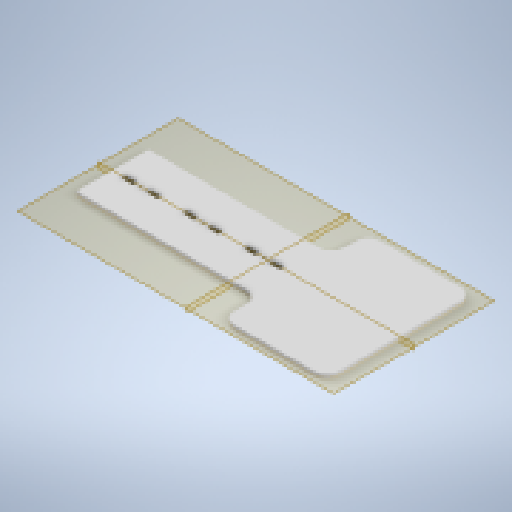
# Autodesk Inventor part: Крепление хвоста
Saved by Autodesk Inventor 2023.2 (Build 272271030, 271C)
## iProperties
Created: 2024-03-15
Part Number: Крепление хвоста
Material: Типовые
Document SubType Name: Modeling
Designer: I9232
Density: 1 g/cm^3
Appearance: По умолчанию
Author: I9232
Autodesk Inventor part; units mm, degrees
sketch "Эскиз1" plane through (0, 0, 0) normal (0, 1, 0) x (-1, 0, 0)
  line L0 (126.566, 29.5) -> (-22.5, 29.5)
  line L1 (-107.5, 29.5) -> (-107.5, -29.5)
  line L2 (-22.5, -29.5) -> (126.566, -29.5)
  line L3 (126.566, -29.5) -> (126.566, 29.5)
  line L4 (-22.5, 29.5) -> (-22.4506, 59.5)
  line L5 (-22.4506, 59.5) -> (-107.4506, 59.5)
  line L6 (-107.4506, 59.5) -> (-107.5, 29.5)
  line L7 (-22.5, -29.5) -> (-22.4506, -59.5)
  line L8 (-22.4506, -59.5) -> (-107.4506, -59.5)
  line L9 (-107.4506, -59.5) -> (-107.5, -29.5)
  point P0 (0, 0)
  dimension "d6" = 59
  dimension "d7" = 119
  dimension "d8" = 149.066
  dimension "d9" = 85
  dimension "d10" = 30
  constraints: 20 end point, 4 parallel, 3 equal length, 1 horizontal, 1 perpendicular, 1 vertical, 2 other
  measures "d6" distance of L2.end L0.start
  measures "d7" distance of L8.end L5.end
  measures "d8" distance of L0.start L0.end
  measures "d9" distance of L4.end L5.end
  measures "d10" distance of L0.end L4.end
extrude "Выдавливание1" add sketch "Эскиз1" along normal mid plane 4
fillet "Сопряжение1" radius 10 6 edges at (22.5, 0, -29.5) (22.4506, 0, -59.5) (22.4506, 0, 59.5) (107.4506, 0, -59.5) (107.4506, 0, 59.5) (22.5, 0, 29.5)
sketch "Эскиз2" plane through (0, -2, 0) normal (0, -1, 0) x (1, 0, 0)
  line L0 (-118.066, -2) -> (-108.066, -2) projected
  line L1 (-108.066, -2) -> (-108.066, 2) projected
  line L2 (-108.066, 2) -> (-118.066, 2) projected
  line L3 (-118.066, 2) -> (-118.066, -2) projected
  line L4 (-98.066, -2) -> (-88.066, -2) projected
  line L5 (-88.066, -2) -> (-88.066, 2) projected
  line L6 (-88.066, 2) -> (-98.066, 2) projected
  line L7 (-98.066, 2) -> (-98.066, -2) projected
  line L8 (-68.066, -2) -> (-58.066, -2) projected
  line L9 (-58.066, -2) -> (-58.066, 2) projected
  line L10 (-58.066, 2) -> (-68.066, 2) projected
  line L11 (-68.066, 2) -> (-68.066, -2) projected
  line L12 (-48.066, -2) -> (-38.066, -2) projected
  line L13 (-38.066, -2) -> (-38.066, 2) projected
  line L14 (-38.066, 2) -> (-48.066, 2) projected
  line L15 (-48.066, 2) -> (-48.066, -2) projected
  line L16 (-18.066, -2) -> (-8.066, -2) projected
  line L17 (-8.066, -2) -> (-8.066, 2) projected
  line L18 (-8.066, 2) -> (-18.066, 2) projected
  line L19 (-18.066, 2) -> (-18.066, -2) projected
  line L20 (1.934, -2) -> (11.934, -2) projected
  line L21 (11.934, -2) -> (11.934, 2) projected
  line L22 (11.934, 2) -> (1.934, 2) projected
  line L23 (1.934, 2) -> (1.934, -2) projected
  point P0 (0, 0)
extrude "Выдавливание2" cut sketch "Эскиз2" against normal up to surface (4 mm away)
sketch "Эскиз3" plane through (0, -2, 0) normal (0, -1, 0) x (1, 0, 0)
  line L0 (1.934, 2) -> (1.934, -2) projected
  line L1 (-8.066, -2) -> (-8.066, 2) projected
  line L2 (-48.066, 2) -> (-48.066, -2) projected
  line L3 (-58.066, -2) -> (-58.066, 2) projected
  line L4 (-98.066, 2) -> (-98.066, -2) projected
  line L5 (-108.066, -2) -> (-108.066, 2) projected
  circle A0 centre (-3.066, 0) radius 1.5
  circle A1 centre (-53.066, 0) radius 1.5
  circle A2 centre (-103.066, 0) radius 1.5
  line L6 (1.934, 2) -> (1.934, -2) projected
  line L7 (1.934, 0) -> (-8.066, 0) construction
  line L8 (-8.066, 2) -> (-8.066, -2) projected
  line L9 (-48.066, -2) -> (-48.066, 2) projected
  line L10 (-48.066, 0) -> (-58.066, 0) construction
  line L11 (-58.066, 2) -> (-58.066, -2) projected
  line L12 (-98.066, -2) -> (-98.066, 2) projected
  line L13 (-98.066, 0) -> (-108.066, 0) construction
  line L14 (-108.066, 2) -> (-108.066, -2) projected
  point P0 (0, 0)
  point P1 (-3.066, 0)
  point P2 (-53.066, 0)
  point P3 (-103.066, 0)
  dimension "d14" = 3
  constraints: 9 midpoint, 6 end point, 3 centre point, 3 coincident, 2 equal radius
  measures "d14" diameter of A0
extrude "Выдавливание3" cut sketch "Эскиз3" against normal up to surface (4 mm away)
sketch "Эскиз4" plane through (-126.566, -2, 29.5) normal (-1, 0, 0) x (0, 0, 1)
  line L0 (0, 4) -> (-59, 4) projected
  line L1 (-59, 0) -> (0, 0) projected
  line L2 (-54.5, 4) -> (-49.5, 4)
  line L3 (-49.5, 4) -> (-49.5, 0)
  line L4 (-49.5, 0) -> (-54.5, 0)
  line L5 (-54.5, 0) -> (-54.5, 4)
  line L6 (-59, 4) -> (-59, 0) projected
  line L7 (-39.5, 4) -> (-34.5, 4)
  line L8 (-34.5, 4) -> (-34.5, 0)
  line L9 (-34.5, 0) -> (-39.5, 0)
  line L10 (-39.5, 0) -> (-39.5, 4)
  line L11 (-24.5, 4) -> (-19.5, 4)
  line L12 (-19.5, 4) -> (-19.5, 0)
  line L13 (-19.5, 0) -> (-24.5, 0)
  line L14 (-24.5, 0) -> (-24.5, 4)
  line L15 (-9.5, 4) -> (-4.5, 4)
  line L16 (-4.5, 4) -> (-4.5, 0)
  line L17 (-4.5, 0) -> (-9.5, 0)
  line L18 (-9.5, 0) -> (-9.5, 4)
  point P0 (-29.5, 2)
  point P1 (-9.5, 0)
  point P2 (-24.5, 0)
  point P3 (-39.5, 0)
  point P4 (-54.5, 0)
  dimension "d17" = 5
  dimension "d18" = 4.5
  dimension "d19" = 10
  dimension "d20" = 5
  dimension "d23" = 30
  constraints: 32 end point, 4 parallel, 4 point on line, 3 horizontal, 2 perpendicular, 16 other
  measures "d17" distance of L2.end L2.start
  measures "d18" distance between parallel lines of L5 L6
  measures "d19" distance between parallel lines of L10 L3
  measures "d20" distance of L8.end L9.end
  measures "d23" distance of L2.start L11.start
extrude "Выдавливание4" add sketch "Эскиз4" along normal blind 3 contours L16 L1 L18 L0 | L12 L1 L14 L0 | L8 L1 L10 L0 | L3 L1 L5 L0
sketch "Эскиз5" plane through (-126.566, -2, -29.5) normal (0, 0, -1) x (-1, 0, 0)
  line L0 (0, 4) -> (-139.0495, 4) projected
  line L1 (-18.5, 0) -> (-8.5, 0) projected
  line L2 (-15, 4) -> (-5, 4)
  line L3 (-5, 4) -> (-5, 0)
  line L4 (-5, 0) -> (-15, 0)
  line L5 (-15, 0) -> (-15, 4)
  line L6 (0, 0) -> (-139.0495, 0) projected
  line L7 (-35, 4) -> (-25, 4)
  line L8 (-25, 4) -> (-25, 0)
  line L9 (-25, 0) -> (-35, 0)
  line L10 (-35, 0) -> (-35, 4)
  line L11 (0, 4) -> (0, 0) projected
  line L12 (-55, 4) -> (-45, 4)
  line L13 (-45, 4) -> (-45, 0)
  line L14 (-45, 0) -> (-55, 0)
  line L15 (-55, 0) -> (-55, 4)
  line L16 (-75, 4) -> (-65, 4)
  line L17 (-65, 4) -> (-65, 0)
  line L18 (-65, 0) -> (-75, 0)
  line L19 (-75, 0) -> (-75, 4)
  point P0 (-126.566, 2)
  point P1 (-15, 0)
  point P2 (-35, 0)
  point P3 (-55, 0)
  point P4 (-75, 0)
  dimension "d30" = 10
  dimension "d31" = 10
  dimension "d32" = 5
  dimension "d33" = 10
  dimension "d36" = 40
  constraints: 32 end point, 5 point on line, 4 parallel, 3 horizontal, 2 perpendicular, 16 other
  measures "d30" distance of L7.end L7.start
  measures "d31" distance of L2.end L2.start
  measures "d32" distance between parallel lines of L11 L3
  measures "d33" distance between parallel lines of L5 L8
  measures "d36" distance of L2.start L12.start
extrude "Выдавливание5" add sketch "Эскиз5" along normal blind 3 contours L3 L4 L1 L5 L0 | L8 L6 L10 L0 | L13 L6 L15 L0 | L17 L6 L19 L0
mirror "Зеркальное отражение1" about plane through (0, 0, 0) normal (0, 0, 1) of "Выдавливание5"
sketch "Эскиз6" plane through (0, -2, 0) normal (0, -1, 0) x (1, 0, 0)
  line L0 (93.0791, -30.9) -> (93.0791, -26.9) projected
  line L1 (93.0791, -26.9) -> (87.0791, -26.9) projected
  line L2 (87.0791, -26.9) -> (87.0791, -30.9) projected
  line L3 (87.0791, -30.9) -> (93.0791, -30.9) projected
  line L4 (93.0791, 30.9) -> (93.0791, 26.9) projected
  line L5 (87.0791, 30.9) -> (93.0791, 30.9) projected
  line L6 (87.0791, 26.9) -> (87.0791, 30.9) projected
  line L7 (93.0791, 26.9) -> (87.0791, 26.9) projected
  line L8 (71.0791, 30.9) -> (77.0791, 30.9) projected
  line L9 (77.0791, 30.9) -> (77.0791, 26.9) projected
  line L10 (77.0791, 26.9) -> (71.0791, 26.9) projected
  line L11 (71.0791, 26.9) -> (71.0791, 30.9) projected
  line L12 (58.5057, 30.9) -> (58.5057, 26.9) projected
  line L13 (58.5057, 26.9) -> (52.5057, 26.9) projected
  line L14 (52.5057, 30.9) -> (58.5057, 30.9) projected
  line L15 (52.5057, 26.9) -> (52.5057, 30.9) projected
  line L16 (42.5057, 30.9) -> (42.5057, 26.9) projected
  line L17 (42.5057, 26.9) -> (36.5057, 26.9) projected
  line L18 (36.5057, 26.9) -> (36.5057, 30.9) projected
  line L19 (36.5057, 30.9) -> (42.5057, 30.9) projected
  line L20 (77.0791, -26.9) -> (71.0791, -26.9) projected
  line L21 (71.0791, -30.9) -> (77.0791, -30.9) projected
  line L22 (77.0791, -30.9) -> (77.0791, -26.9) projected
  line L23 (71.0791, -26.9) -> (71.0791, -30.9) projected
  line L24 (58.5057, -30.9) -> (58.5057, -26.9) projected
  line L25 (52.5057, -30.9) -> (58.5057, -30.9) projected
  line L26 (58.5057, -26.9) -> (52.5057, -26.9) projected
  line L27 (52.5057, -26.9) -> (52.5057, -30.9) projected
  line L28 (42.5057, -30.9) -> (42.5057, -26.9) projected
  line L29 (36.5057, -30.9) -> (42.5057, -30.9) projected
  line L30 (42.5057, -26.9) -> (36.5057, -26.9) projected
  line L31 (36.5057, -26.9) -> (36.5057, -30.9) projected
  point P0 (0, 0)
extrude "Выдавливание6" cut sketch "Эскиз6" against normal up to surface (4 mm away)
sketch "Эскиз7" plane through (0, -2, 0) normal (0, -1, 0) x (1, 0, 0)
  point P0 (0, 0)
sketch "Эскиз8" plane through (0, -2, 0) normal (0, -1, 0) x (1, 0, 0)
  circle A0 centre (82.0791, -28.9) radius 1.5
  circle A1 centre (82.0791, 28.9) radius 1.5
  circle A2 centre (47.5057, 28.9) radius 1.5
  circle A3 centre (47.5057, -28.9) radius 1.5
  line L0 (52.5057, -30.9) -> (52.5057, -26.9) projected
  line L1 (42.5057, -26.9) -> (42.5057, -30.9) projected
  line L2 (77.0791, -26.9) -> (77.0791, -30.9) projected
  line L3 (87.0791, -26.9) -> (87.0791, -30.9) projected
  line L4 (87.0791, 26.9) -> (87.0791, 30.9) projected
  line L5 (77.0791, 30.9) -> (77.0791, 26.9) projected
  line L6 (52.5057, 26.9) -> (52.5057, 30.9) projected
  line L7 (42.5057, 30.9) -> (42.5057, 26.9) projected
  line L8 (87.0791, -26.9) -> (87.0791, -30.9) projected
  line L9 (87.0791, -28.9) -> (77.0791, -28.9) construction
  line L10 (77.0791, -30.9) -> (77.0791, -26.9) projected
  line L11 (52.5057, -28.9) -> (42.5057, -28.9) construction
  line L12 (87.0791, 26.9) -> (87.0791, 30.9) projected
  line L13 (87.0791, 28.9) -> (77.0791, 28.9) construction
  line L14 (52.5057, 28.9) -> (42.5057, 28.9) construction
  point P0 (0, 0)
  point P1 (82.0791, -28.9)
  point P2 (47.5057, 28.9)
  point P3 (82.0791, 28.9)
  dimension "d45" = 3
  constraints: 12 midpoint, 8 end point, 4 centre point, 4 coincident, 3 equal radius
  measures "d45" diameter of A0
extrude "Выдавливание7" cut sketch "Эскиз8" against normal up to surface (4 mm away)
sketch "Эскиз9" plane through (0, 2, 0) normal (0, 1, 0) x (1, 0, 0)
  line L0 (-108.016, -29.5) -> (-105.116, -29.5)
  line L1 (-105.116, -14.6) -> (-108.016, -14.6)
  line L2 (-111.566, -29.5) -> (-101.566, -29.5) projected
  line L3 (-103.766, -21.4) -> (-103.766, -19.6)
  line L4 (-109.366, -19.6) -> (-109.366, -21.4)
  line L5 (-106.566, -14.6) -> (-106.566, -29.5) construction
  line L6 (-108.016, -14.6) -> (-108.016, -19.6)
  line L7 (-108.016, -21.4) -> (-108.016, -29.5)
  line L8 (-109.366, -21.4) -> (-108.016, -21.4)
  line L9 (-105.116, -21.4) -> (-103.766, -21.4)
  line L10 (-103.766, -19.6) -> (-105.116, -19.6)
  line L11 (-108.016, -19.6) -> (-109.366, -19.6)
  line L12 (-105.116, -29.5) -> (-105.116, -21.4)
  line L13 (-105.116, -19.6) -> (-105.116, -14.6)
  line L14 (-68.016, -19.6) -> (-69.366, -19.6)
  line L15 (-68.016, -14.6) -> (-68.016, -19.6)
  line L16 (-65.116, -19.6) -> (-65.116, -14.6)
  line L17 (-65.116, -14.6) -> (-68.016, -14.6)
  line L18 (-69.366, -21.4) -> (-68.016, -21.4)
  line L19 (-69.366, -19.6) -> (-69.366, -21.4)
  line L20 (-63.766, -21.4) -> (-63.766, -19.6)
  line L21 (-65.116, -21.4) -> (-63.766, -21.4)
  line L22 (-66.566, -14.6) -> (-66.566, -29.5) construction
  line L23 (-68.016, -21.4) -> (-68.016, -29.5)
  line L24 (-65.116, -29.5) -> (-65.116, -21.4)
  line L25 (-68.016, -29.5) -> (-65.116, -29.5)
  line L26 (-63.766, -19.6) -> (-65.116, -19.6)
  line L27 (-94.5323, 0) -> (-86.001, 0) construction
  line L28 (-108.016, 29.5) -> (-105.116, 29.5)
  line L29 (-105.116, 14.6) -> (-108.016, 14.6)
  line L30 (-111.566, 29.5) -> (-101.566, 29.5)
  line L31 (-103.766, 21.4) -> (-103.766, 19.6)
  line L32 (-109.366, 19.6) -> (-109.366, 21.4)
  line L33 (-106.566, 14.6) -> (-106.566, 29.5) construction
  line L34 (-108.016, 14.6) -> (-108.016, 19.6)
  line L35 (-108.016, 21.4) -> (-108.016, 29.5)
  line L36 (-109.366, 21.4) -> (-108.016, 21.4)
  line L37 (-105.116, 21.4) -> (-103.766, 21.4)
  line L38 (-103.766, 19.6) -> (-105.116, 19.6)
  line L39 (-108.016, 19.6) -> (-109.366, 19.6)
  line L40 (-105.116, 29.5) -> (-105.116, 21.4)
  line L41 (-105.116, 19.6) -> (-105.116, 14.6)
  line L42 (-68.016, 19.6) -> (-69.366, 19.6)
  line L43 (-68.016, 14.6) -> (-68.016, 19.6)
  line L44 (-65.116, 19.6) -> (-65.116, 14.6)
  line L45 (-65.116, 14.6) -> (-68.016, 14.6)
  line L46 (-69.366, 21.4) -> (-68.016, 21.4)
  line L47 (-69.366, 19.6) -> (-69.366, 21.4)
  line L48 (-63.766, 21.4) -> (-63.766, 19.6)
  line L49 (-65.116, 21.4) -> (-63.766, 21.4)
  line L50 (-66.566, 14.6) -> (-66.566, 29.5) construction
  line L51 (-68.016, 21.4) -> (-68.016, 29.5)
  line L52 (-65.116, 29.5) -> (-65.116, 21.4)
  line L53 (-68.016, 29.5) -> (-65.116, 29.5)
  line L54 (-63.766, 19.6) -> (-65.116, 19.6)
  line L55 (-126.566, -10) -> (-126.566, -20) projected
  line L56 (-116.566, -16.45) -> (-116.566, -13.55)
  line L57 (-126.566, -13.55) -> (-126.566, -16.45)
  line L58 (-121.566, -17.8) -> (-119.766, -17.8)
  line L59 (-119.766, -12.2) -> (-121.566, -12.2)
  line L60 (-116.566, -15) -> (-126.566, -15) construction
  line L61 (-126.566, 10) -> (-126.566, 20)
  line L62 (-116.566, 16.45) -> (-116.566, 13.55)
  line L63 (-126.566, 13.55) -> (-126.566, 16.45)
  line L64 (-121.566, 17.8) -> (-119.766, 17.8)
  line L65 (-119.766, 12.2) -> (-121.566, 12.2)
  line L66 (-116.566, 15) -> (-126.566, 15) construction
  line L67 (-121.566, -12.2) -> (-121.566, -13.55)
  line L68 (-121.566, -16.45) -> (-121.566, -17.8)
  line L69 (-119.766, -17.8) -> (-119.766, -16.45)
  line L70 (-119.766, -13.55) -> (-119.766, -12.2)
  line L71 (-126.566, -16.45) -> (-121.566, -16.45)
  line L72 (-119.766, -16.45) -> (-116.566, -16.45)
  line L73 (-116.566, -13.55) -> (-119.766, -13.55)
  line L74 (-121.566, -13.55) -> (-126.566, -13.55)
  line L75 (-116.566, 13.55) -> (-119.766, 13.55)
  line L76 (-121.566, 13.55) -> (-126.566, 13.55)
  line L77 (-121.566, 12.2) -> (-121.566, 13.55)
  line L78 (-121.566, 16.45) -> (-121.566, 17.8)
  line L79 (-119.766, 17.8) -> (-119.766, 16.45)
  line L80 (-119.766, 13.55) -> (-119.766, 12.2)
  line L81 (-126.566, 16.45) -> (-121.566, 16.45)
  line L82 (-119.766, 16.45) -> (-116.566, 16.45)
  point P0 (0, 0)
  point P1 (-104.441, -19.6)
  point P2 (-108.691, -21.4)
  point P3 (-64.441, -19.6)
  point P4 (-68.691, -21.4)
  point P5 (-104.441, 19.6)
  point P6 (-108.691, 21.4)
  point P7 (-64.441, 19.6)
  point P8 (-68.691, 21.4)
  point P9 (-121.566, -15)
  point P10 (-121.566, 15)
  dimension "d48" = 2.9
  dimension "d49" = 1.8
  dimension "d50" = 5.6
  dimension "d52" = 1.35
  dimension "d53" = 5
  dimension "d54" = 8.1
  dimension "d55" = 8.1
  dimension "d58" = 40
  dimension "d63" = 10
  dimension "d64" = 2.9
  dimension "d65" = 1.8
  dimension "d66" = 5.6
  dimension "d68" = 1.35
  constraints: 162 end point, 47 symmetric about line, 20 parallel, 11 equal length, 10 midpoint, 10 perpendicular, 8 horizontal, 2 point on line, 29 other
  measures "d48" distance of L1.start L1.end
  measures "d49" distance of L4.start L4.end
  measures "d50" distance of L3.end L4.start
  measures "d52" distance of L6.end L4.start
  measures "d53" vertical distance of L1.start point (-104.441, -19.6)
  measures "d54" distance from line of L0 point (-108.691, -21.4)
  measures "d55" distance between parallel lines of L2 L9
  measures "d58" distance of point (-104.441, -19.6) point (-64.441, -19.6)
  measures "d63" distance of L57.end L56.start
  measures "d64" distance of L56.start L56.end
  measures "d65" distance of L59.start L59.end
  measures "d66" distance of L58.end L59.start
  measures "d68" distance of L70.start L59.start
extrude "Выдавливание8" cut sketch "Эскиз9" against normal up to surface (4 mm away)
